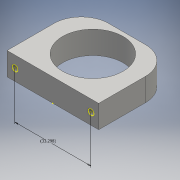
# Autodesk Inventor part: motor holder
Saved by Autodesk Inventor 2016 (Build 200138000, 138)
## iProperties
Created: 2017-07-15
Part Number: motor holder
Material: Generic
Document SubType Name: Modeling
Designer: ALIREZA
Density: 1 g/cm^3
Appearance: Default
Author: ALIREZA
Autodesk Inventor part; units mm, degrees
ref_plane "YZ Plane" through (0, 0, 0) normal (1, 0, 0) x (0, 1, 0)
ref_plane "XZ Plane" through (0, 0, 0) normal (0, 1, 0) x (-1, 0, 0)
ref_plane "XY Plane" through (0, 0, 0) normal (0, 0, 1) x (1, 0, 0)
sketch "Sketch1" plane through (0, 0, 0) normal (0, 0, 1) x (1, 0, 0)
  line L0 (16, -17.5) -> (16, 15)
  line L1 (-16, 15) -> (-16, -17.5)
  circle A0 centre (0, 0) radius 13.25
  line L2 (16, -17.5) -> (-16, -17.5)
  line L3 (-16, -17.5) -> (-16, 15)
  line L4 (16, 15) -> (-16, 15)
  dimension "d2" = 26.5
  dimension "d4" = 17.5
  dimension "d5" = 32.5
  constraints: 10 end point, 2 perpendicular, 1 centre point, 1 coincident, 1 parallel
  measures "d2" diameter of A0
  measures "d4" distance from line of L2 point (0, 0)
  measures "d5" distance between parallel lines of L4 L2
extrude "Extrusion1" add sketch "Sketch1" along normal blind 10
sketch "Sketch2" plane through (0, 0, 0) normal (0, 0, -1) x (-1, 0, 0)
  point P0 (0, 0)
sketch "Sketch3" plane through (0, 0, 0) normal (0, 0, -1) x (-1, 0, 0)
  line L0 (16, 15) -> (16, -17.5) projected
  line L1 (17.8498, -17.5) -> (20.048, -17.5)
  line L2 (20.048, -17.5) -> (20.048, 15)
  line L3 (20.048, 15) -> (16, 15)
  line L4 (-16, 15) -> (16, 15) projected
  line L5 (16, -17.5) -> (16, 15)
  line L6 (0, 0) -> (0, 7.3422)
  line L7 (-16, 15) -> (-16, -17.5)
  line L8 (-17.8498, -17.5) -> (-20.048, -17.5)
  line L9 (-20.048, -17.5) -> (-20.048, 15)
  line L10 (-20.048, 15) -> (-16, 15)
  line L11 (17.8498, -17.5) -> (16, -17.5)
  line L12 (16, 15) -> (16, -17.5) projected
  line L13 (20.048, 15) -> (16, 15)
  line L14 (16, -17.5) -> (-16, -17.5) projected
  line L15 (-17.8498, -17.5) -> (-16, -17.5)
  constraints: 24 end point, 3 perpendicular, 3 symmetric about line, 2 horizontal, 2 vertical, 1 collinear
extrude "Extrusion2" add sketch "Sketch3" against normal up to surface (10 mm away) contours L3 L2 L1 L11 L0 | L7 L15 L8 L9 L10
sketch "Sketch4" plane through (-20.048, -17.5, 0) normal (0, -1, 0) x (1, 0, 0)
  line L0 (40.0961, 0) -> (0, 0) projected
  line L1 (40.0961, 10) -> (0, 10) projected
  circle A0 centre (3.399, 5) radius 1.25
  circle A1 centre (36.697, 5) radius 1.25
  point P0 (20.048, 0)
  dimension "d11" = 2.5
  constraints: 2 centre point
  measures "d11" diameter of A0
extrude "Extrusion3" cut sketch "Sketch4" against normal blind 27
fillet "Fillet1" radius 12 2 edges at (20.048, 15, 5) (-20.048, 15, 5)
sketch "Sketch5" plane through (-20.048, -17.5, 0) normal (0, -1, 0) x (1, 0, 0)
  circle A0 centre (3.399, 5) radius 1.25 projected
  circle A1 centre (36.697, 5) radius 1.25 projected
  point P0 (20.048, 0)
  dimension "d15" = 33.298
  measures "d15" distance of A1.centre A0.centre
body "Solid1"
